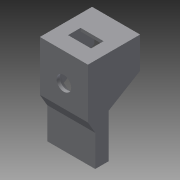
# Autodesk Inventor part: anti_axe_2
Saved by Autodesk Inventor 2014 SP1 (Build 180222100, 222)
## iProperties
Created: 2015-02-02
Part Number: anti_axe_2
Material: Générique
Document SubType Name: Modeling
Designer: astralien3000
Density: 1 g/cm^3
Appearance: Par défaut
Author: astralien3000
Autodesk Inventor part; units mm, degrees
ref_plane "YZ Plane" through (0, 0, 0) normal (1, 0, 0) x (0, 1, 0)
ref_plane "XZ Plane" through (0, 0, 0) normal (0, 1, 0) x (-1, 0, 0)
ref_plane "XY Plane" through (0, 0, 0) normal (0, 0, 1) x (1, 0, 0)
sketch "Esquisse1" plane through (0, 0, 0) normal (0, 1, 0) x (-1, 0, 0)
  line L0 (-10.5, 21) -> (10.5, 21)
  line L1 (10.5, 21) -> (10.5, -21)
  line L2 (10.5, -21) -> (-10.5, -21)
  line L3 (-10.5, -21) -> (-10.5, 21)
  line L4 (10.5, -21) -> (11.5, -21)
  line L5 (11.5, -21) -> (11.5, 21)
  line L6 (11.5, 21) -> (10.5, 21)
  line L7 (10.5, 21) -> (10.5, -21)
  line L8 (-10.5, 21) -> (-11.5, 21)
  line L9 (-11.5, 21) -> (-11.5, -21)
  line L10 (-11.5, -21) -> (-10.5, -21)
  line L11 (-10.5, -21) -> (-10.5, 21)
  line L12 (11.5, 21) -> (-11.5, 21)
  line L13 (-11.5, 21) -> (-11.5, 22.5)
  line L14 (-11.5, 22.5) -> (11.5, 22.5)
  line L15 (11.5, 22.5) -> (11.5, 21)
  line L16 (11.5, -21) -> (-11.5, -21)
  line L17 (-11.5, -21) -> (-11.5, -22.5)
  line L18 (-11.5, -22.5) -> (11.5, -22.5)
  line L19 (11.5, -22.5) -> (11.5, -21)
  point P0 (0, 0)
  dimension "d0" = 21
  dimension "d1" = 42
  dimension "d2" = 21
  dimension "d3" = 10.5
  dimension "d4" = 1
  dimension "d5" = 1
  dimension "d6" = 1.5
  dimension "d7" = 1.5
  constraints: 40 end point, 10 parallel, 5 horizontal, 5 perpendicular, 3 collinear
  measures "d0" distance between parallel lines of L11 L7
  measures "d1" distance between parallel lines of L2 L0
  measures "d2" distance from line of point (0, 0) L0
  measures "d3" distance from line of point (0, 0) L7
  measures "d4" distance between parallel lines of L9 L11
  measures "d5" distance between parallel lines of L7 L5
  measures "d6" distance between parallel lines of L0 L14
  measures "d7" distance between parallel lines of L2 L18
extrude "Extrusion1" add sketch "Esquisse1" along normal blind 5
sketch "Esquisse2" plane through (0, 5, 0) normal (0, 1, 0) x (1, 0, 0)
  line L0 (11.5, -22.5) -> (11.5, 22.5) projected
  line L1 (11.5, 22.5) -> (-11.5, 22.5) projected
  line L2 (-11.5, 22.5) -> (-11.5, -22.5) projected
  line L3 (-11.5, -22.5) -> (11.5, -22.5) projected
  line L4 (-10.5, 21) -> (10.5, 21)
  line L5 (10.5, 21) -> (10.5, -21)
  line L6 (10.5, -21) -> (-10.5, -21)
  line L7 (-10.5, -21) -> (-10.5, 21)
  point P0 (0, 0)
  dimension "d10" = 1
  dimension "d11" = 1
  dimension "d12" = 1.5
  dimension "d13" = 1.5
  constraints: 8 end point, 2 parallel, 1 horizontal, 1 perpendicular
  measures "d10" distance between parallel lines of L0 L5
  measures "d11" distance between parallel lines of L2 L7
  measures "d12" distance between parallel lines of L1 L4
  measures "d13" distance between parallel lines of L3 L6
extrude "Extrusion2" add sketch "Esquisse2" along normal blind 20
sketch "Esquisse3" plane through (0, 5, 0) normal (0, 1, 0) x (1, 0, 0)
  line L0 (10.5, -21) -> (10.5, 21) projected
  line L1 (-10.5, 21) -> (-10.5, -21) projected
  line L2 (10.5, -21) -> (0, -21)
  line L3 (0, -21) -> (0, -9) construction
  line L4 (0, -9) -> (10.5, -9) construction
  line L5 (10.5, -9) -> (10.5, -21)
  circle A0 centre (0, -9) radius 3.5
  point P0 (0, 0)
  dimension "d16" = 12
  dimension "d17" = 10.5
  dimension "d18" = 21
  dimension "d19" = 7
  constraints: 8 end point, 2 parallel, 1 centre point, 1 coincident, 1 horizontal, 1 perpendicular
  measures "d16" distance of L2.end L3.end
  measures "d17" distance between parallel lines of L1 L3
  measures "d18" distance between parallel lines of L0 L1
  measures "d19" diameter of A0
extrude "Extrusion3" cut sketch "Esquisse3" against normal through all
sketch "Esquisse4" plane through (-11.5, 0, -22.5) normal (-1, 0, 0) x (0, 0, 1)
  line L0 (45, 0) -> (45, 25) projected
  line L1 (0, 25) -> (21, 25)
  line L2 (21, 25) -> (21, 10) construction
  line L3 (21, 10) -> (0, 10)
  line L4 (0, 10) -> (0, 25)
  line L5 (45, 25) -> (30, 25)
  line L6 (30, 25) -> (30, 10) construction
  line L7 (30, 10) -> (45, 10) construction
  line L8 (45, 10) -> (45, 25)
  line L9 (21, 10) -> (30, 25)
  line L10 (30, 25) -> (21, 25)
  point P0 (22.5, 0)
  dimension "d22" = 15
  dimension "d23" = 24
  dimension "d24" = 15
  constraints: 20 end point, 4 parallel, 3 perpendicular, 2 horizontal, 1 collinear
  measures "d22" distance between parallel lines of L1 L3
  measures "d23" distance between parallel lines of L0 L2
  measures "d24" distance between parallel lines of L8 L6
extrude "Extrusion4" cut sketch "Esquisse4" against normal through all
sketch "Esquisse5" plane through (-11.5, 0, -22.5) normal (-1, 0, 0) x (0, 0, 1)
  line L0 (0, 0) -> (45, 0) projected
  line L1 (45, 0) -> (45, 25) projected
  line L2 (0, 0) -> (15, 0)
  line L3 (15, 0) -> (15, 3.5) construction
  line L4 (15, 3.5) -> (0, 3.5)
  line L5 (0, 3.5) -> (0, 0)
  line L6 (45, 0) -> (21, 0)
  line L7 (21, 0) -> (21, 3.5) construction
  line L8 (21, 3.5) -> (45, 3.5) construction
  line L9 (45, 3.5) -> (45, 0)
  line L10 (15, 3.5) -> (21, 0)
  line L11 (15, 0) -> (21, 0)
  point P0 (22.5, 0)
  dimension "d27" = 3.5
  dimension "d28" = 30
  dimension "d29" = 24
  constraints: 20 end point, 4 parallel, 3 perpendicular, 2 horizontal, 1 collinear
  measures "d27" distance between parallel lines of L0 L4
  measures "d28" distance between parallel lines of L1 L3
  measures "d29" distance between parallel lines of L1 L7
extrude "Extrusion5" cut sketch "Esquisse5" against normal through all
chamfer "Chanfrein1" distance 3.5 angle 45 1 edges at (-3.5, 5, 9)
sketch "Esquisse8" plane through (10.5, 5, 21) normal (0, 0, -1) x (-1, 0, 0)
  line L0 (21, 0) -> (0, 0) projected
  line L1 (21, 0) -> (21, 20) projected
  line L2 (0, 0) -> (0, 20) projected
  line L3 (5, 8.5) -> (16, 8.5)
  line L4 (16, 8.5) -> (16, 2.5)
  line L5 (16, 2.5) -> (5, 2.5)
  line L6 (5, 2.5) -> (5, 8.5)
  point P0 (10.5, -5)
  dimension "d38" = 2.5
  dimension "d39" = 6
  dimension "d40" = 11
  dimension "d41" = 21
  dimension "d42" = 5
  constraints: 8 end point, 2 parallel, 1 horizontal, 1 perpendicular
  measures "d38" distance between parallel lines of L0 L5
  measures "d39" distance of L3.end L4.end
  measures "d40" distance of L4.end L5.end
  measures "d41" distance between parallel lines of L1 L2
  measures "d42" distance between parallel lines of L1 L4
extrude "Extrusion6" cut sketch "Esquisse8" against normal through all
equation "\"d2\" = 0.5 * d1"
equation "\"d3\" = 0.5 * d0"
equation "\"d5\" = d4"
equation "\"d7\" = d6"
equation "\"d11\" = d10"
equation "\"d13\" = d12"
equation "\"d17\" = 0.5 * d18"
equation "\"d42\" = -0.5 * d40 + 0.5 * d41"
